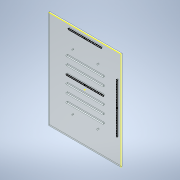
# Autodesk Inventor part: Base
Saved by Autodesk Inventor 2021 (Build 250183000, 183)
## iProperties
Created: 2022-03-22
Part Number: Base
Material: Vidro
Document SubType Name: Modeling
Designer: aluno
Density: 2.18 g/cm^3
Appearance: Transparente
Mass: 817.5 g
Surface Area: 1555 cm^2
Volume: 375 cm^3
Author: aluno
Autodesk Inventor part; units mm, degrees
note: some values were not read from the file. Chosen so that the rebuilt part matches the saved one: direction of "Furo1".
ref_plane "YZ Plane" through (0, 0, 0) normal (1, 0, 0) x (0, 1, 0)
ref_plane "XZ Plane" through (0, 0, 0) normal (0, 1, 0) x (-1, 0, 0)
ref_plane "XY Plane" through (0, 0, 0) normal (0, 0, 1) x (1, 0, 0)
sketch "Esboço1" plane through (0, 0, 0) normal (0, 0, 1) x (1, 0, 0)
  line L0 (-89, -121) -> (89, -121)
  line L1 (89, -121) -> (89, 121)
  line L2 (89, 121) -> (-89, 121)
  line L3 (-89, 121) -> (-89, -121)
  line L4 (-89, -121) -> (89, 121) construction
  line L5 (89, -121) -> (-89, 121) construction
  point P0 (0, 0)
  dimension "d0" = 178
  dimension "d1" = 242
  constraints: 12 end point, 2 midpoint, 2 parallel, 1 horizontal, 1 perpendicular
  measures "d0" distance of L1.end L2.end
  measures "d1" distance of L2.end L0.start
extrude "Extrusão1" add sketch "Esboço1" along normal blind 3
sketch "Esboço2" plane through (0, 0, 3) normal (0, 0, 1) x (1, 0, 0)
  circle A0 centre (-31, 69.5) radius 1.2295 projected
  circle A1 centre (31, 69.5) radius 1.2295 projected
  circle A2 centre (-31, -69.5) radius 1.2295 projected
  circle A3 centre (31, -69.5) radius 1.2295 projected
  point P0 (0, 0)
hole "Furo1" at (-31, 69.5, 3) at (31, 69.5, 3) at (-31, -69.5, 3) at (31, -69.5, 3) direction (0, 0, -1) diameter 3 depth 3
sketch "Esboço3" plane through (0, 0, 3) normal (0, 0, 1) x (1, 0, 0)
  line L0 (-40, 110) -> (40, 110) construction
  line L1 (-40, 108.5) -> (40, 108.5)
  line L2 (40, 111.5) -> (-40, 111.5)
  arc A0 (-40, 111.5) -> (-40, 108.5) centre (-40, 110) ccw
  arc A1 (40, 108.5) -> (40, 111.5) centre (40, 110) ccw
  line L3 (89, 121) -> (-89, 121) projected
  line L4 (79, 60) -> (79, -60) construction
  line L5 (77.5, 60) -> (77.5, -60)
  line L6 (80.5, -60) -> (80.5, 60)
  arc A2 (80.5, 60) -> (77.5, 60) centre (79, 60) ccw
  arc A3 (77.5, -60) -> (80.5, -60) centre (79, -60) ccw
  line L7 (89, -121) -> (89, 121) projected
  line L8 (-45, 10) -> (45, 10) construction
  line L9 (-45, 8.5) -> (45, 8.5)
  line L10 (45, 11.5) -> (-45, 11.5)
  arc A4 (-45, 11.5) -> (-45, 8.5) centre (-45, 10) ccw
  arc A5 (45, 8.5) -> (45, 11.5) centre (45, 10) ccw
  point P0 (0, 0)
  point P1 (0, 110)
  point P2 (79, 0)
  point P3 (0, 10)
  dimension "d11" = 80
  dimension "d12" = 3
  dimension "d20" = 120
  dimension "d21" = 3
  dimension "d22" = 10
  dimension "d23" = 90
  dimension "d24" = 3
  dimension "d26" = 10
  dimension "d27" = 110
  constraints: 24 end point, 12 point on circle, 12 tangent, 6 centre point, 3 midpoint, 3 parallel, 2 horizontal, 2 vertical alignment, 1 horizontal alignment, 1 vertical
  measures "d11" distance of L0.start L0.end
  measures "d12" diameter of A1
  measures "d20" distance of L4.start L4.end
  measures "d21" diameter of A3
  measures "d22" distance from line of L7 point (79, 0)
  measures "d23" distance of L8.start L8.end
  measures "d24" diameter of A5
  measures "d26" distance of point (0, 10) point (0, 0)
  measures "d27" distance of point (0, 0) point (0, 110)
extrude "Extrusão2" cut sketch "Esboço3" against normal through all contours A0 L2 A1 L1
extrude "Extrusão4" cut sketch "Esboço3" against normal through all contours A4 L10 A5 L9
extrude "Extrusão5" cut sketch "Esboço3" against normal through all contours A2 L6 A3 L5
pattern_linear "Padrão retangular1" count 6 spacing 20 along (0, -1, 0) of "Extrusão4" first direction both ways yes
pattern_linear "Padrão retangular2" count 2 spacing 20 along (-1, 0, 0) of "Extrusão5"
pattern_linear "Padrão retangular3" count 2 spacing 20 along (0, -1, 0) of "Extrusão2"
pattern_circular "Padrão circular1" count 2 over 360 about axis through (0, 0, -10) along (0, 0, 1) of "Extrusão2", "Padrão retangular3", "Extrusão5", "Padrão retangular2"
